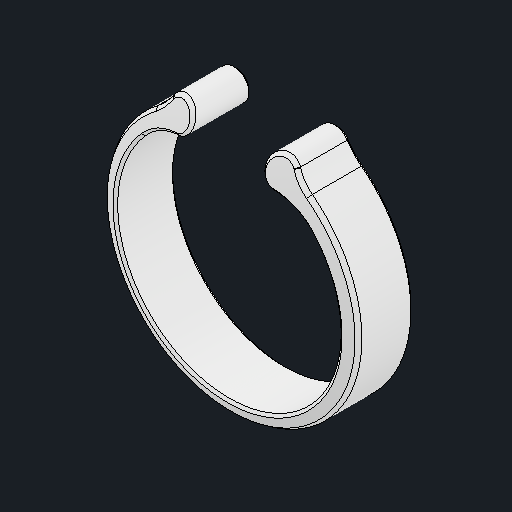
# Autodesk Inventor part: glue-support-port
Saved by Autodesk Inventor 2026 (Build 300175050, 175E)
## iProperties
Created: 2026-01-07
Part Number: glue-support-port
Material: ABS Plastic
Document SubType Name: Modeling
Designer: queezz
Density: 1.06 g/cm^3
Appearance: Smooth - White
Author: queezz
Autodesk Inventor part; units mm, degrees
ref_plane "YZ Plane" through (0, 0, 0) normal (1, 0, 0) x (0, 1, 0)
ref_plane "XZ Plane" through (0, 0, 0) normal (0, 1, 0) x (-1, 0, 0)
ref_plane "XY Plane" through (0, 0, 0) normal (0, 0, 1) x (1, 0, 0)
sketch "Sketch1" plane through (0, 0, 0) normal (0, 0, 1) x (1, 0, 0)
  circle A0 centre (0, 0) radius 42.5
  circle A1 centre (0, 0) radius 37.5
  dimension "d0" = 75
  dimension "d1" = 5
  constraints: 2 centre point, 2 coincident
  measures "d0" diameter of A1
  measures "d1" radial gap between concentric circles of A1 A0
extrude "Extrusion1" add sketch "Sketch1" along normal blind 24
sketch "Sketch2" plane through (0, 0, 24) normal (0, 0, 1) x (1, 0, 0)
  line L0 (0, 0) -> (-29.5833, 63.4415)
  line L1 (-29.5833, 63.4415) -> (29.5833, 63.4415)
  line L2 (29.5833, 63.4415) -> (0, 0)
  dimension "d4" = 50
  dimension "d5" = 70
  constraints: 6 end point, 1 equal length, 1 horizontal
  measures "d4" angle of L0 L2
  measures "d5" distance of L1.end L0.start
extrude "Extrusion2" cut sketch "Sketch2" against normal through all
sketch "Sketch3" plane through (0, 0, 24) normal (0, 0, 1) x (1, 0, 0)
  line L0 (-15.8482, 33.9865) -> (-17.9613, 38.5181) projected
  circle A0 centre (-16.9047, 36.2523) radius 5
  line L1 (15.8482, 33.9865) -> (17.9613, 38.5181) projected
  circle A1 centre (16.9047, 36.2523) radius 5
  point P0 (0, 0)
  dimension "d8" = 10
  constraints: 2 centre point, 2 midpoint, 1 equal radius
  measures "d8" diameter of A0
extrude "Extrusion3" add sketch "Sketch3" against normal up to surface (24 mm away)
fillet "Fillet1" radius 20 4 edges at (-19.543, 32.005, 12) (19.543, 32.005, 12) (21.9019, 36.422, 12) (-21.9019, 36.422, 12)
sketch "Sketch4" plane through (0, 0, 0) normal (1, 0, 0) x (0, 1, 0)
  circle A0 centre (0, -83) radius 110
  line L0 (-37.5, 0) -> (24.7162, 0) projected
  circle A1 centre (0, -83) radius 130
  line L1 (0, 47) -> (0, -213)
  point P0 (0, 0)
  point P1 (0, 27)
  point P2 (0, -193)
  dimension "d15" = 220
  dimension "d16" = 83
  dimension "d17" = 20
  constraints: 2 centre point, 2 end point, 2 point on circle, 1 coincident, 1 vertical, 1 vertical alignment
  measures "d15" diameter of A0
  measures "d16" distance from line of L0 A0.centre
  measures "d17" radial gap between concentric circles of A1 A0
revolve "Revolution1" cut sketch "Sketch4" angle 360 about axis through (0, 0, 47) along (0, 0, -1) picked at (-5.2233, -206.0174) contours A0 L1 A1
chamfer "Chamfer1" distance 1 angle 45 19 edges at (0, -42.5, 0) (23.2765, 36.1041, 0) (12.7211, 38.9904, 0) (22.7626, 29.0787, 0) (0, -37.5, 0) (-22.7626, 29.0787, 0) (-12.7211, 38.9904, 0) (-23.2765, 36.1041, 0) (35.0986, 13.2036, 20.4106) (-34.1548, -15.4822, 20.4106) (22.7578, 29.0813, 20.6164) (12.6875, 38.9384, 19.0922) (23.2743, 36.1066, 18.2651) (38.119, 18.7934, 18.4581) (-40.2431, -13.6655, 18.4581) (-23.2743, 36.1066, 18.2651) (-13.045, 33.0739, 21.0958) (-15.238, 40.9663, 17.9434) (-22.7578, 29.0813, 20.6164)
body "Solid1"
